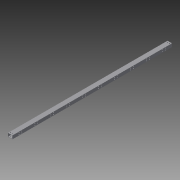
# Autodesk Inventor part: Part1
Saved by Autodesk Inventor 2015 SP1 (Build 190203100, 203)
## iProperties
Created: 2015-03-28
Part Number: Part1
Material: Generic
Document SubType Name: Modeling
Designer: Cyril
Density: 1 g/cm^3
Appearance: Default
Author: Cyril
Autodesk Inventor part; units mm, degrees
ref_plane "YZ Plane" through (0, 0, 0) normal (1, 0, 0) x (0, 1, 0)
ref_plane "XZ Plane" through (0, 0, 0) normal (0, 1, 0) x (-1, 0, 0)
ref_plane "XY Plane" through (0, 0, 0) normal (0, 0, 1) x (1, 0, 0)
sketch "Sketch2" plane through (0, 0, 0) normal (0, 0, 1) x (1, 0, 0)
  line L0 (-18, -13) -> (18, -13)
  line L1 (18, -13) -> (18, 13)
  line L2 (18, 13) -> (-18, 13)
  line L3 (-18, 13) -> (-18, -13)
  line L4 (-17.4388, -13.0791) -> (28.6637, 21.4978) construction
  line L5 (18, -13) -> (-25.5523, 18.4544) construction
  line L6 (-20, -15) -> (20, -15)
  line L7 (20, -15) -> (20, 15)
  line L8 (20, 15) -> (-20, 15)
  line L9 (-20, 15) -> (-20, -15)
  line L10 (-20, -15) -> (20, 15) construction
  line L11 (20, -15) -> (-20, 15) construction
  point P0 (0, 0)
  dimension "d0" = 40
  dimension "d1" = 30
  dimension "d3" = 2
  dimension "d6" = 2
  dimension "d7" = 2
  dimension "d8" = 2
  constraints: 24 end point, 4 parallel, 3 point on line, 2 horizontal, 2 midpoint, 2 perpendicular
  measures "d0" distance of L7.end L8.end
  measures "d1" distance of L8.end L6.start
  measures "d3" distance between parallel lines of L9 L3
  measures "d6" distance between parallel lines of L8 L2
  measures "d7" distance between parallel lines of L7 L1
  measures "d8" distance between parallel lines of L6 L0
extrude "Extrusion1" add sketch "Sketch2" along normal mid plane 1430
sketch "Sketch3" plane through (-20, -15, 715) normal (-1, 0, 0) x (0, 0, 1)
  circle A0 centre (-84, 22.5) radius 3.5
  circle A1 centre (-59, 22.5) radius 3.5
  circle A2 centre (-84, 7.5) radius 3.5
  circle A3 centre (-59, 7.5) radius 3.5
  line L0 (0, 0) -> (-1430, 0) projected
  circle A4 centre (-227, 22.5) radius 3.5
  circle A5 centre (-202, 22.5) radius 3.5
  circle A6 centre (-227, 7.5) radius 3.5
  circle A7 centre (-202, 7.5) radius 3.5
  circle A8 centre (-370, 22.5) radius 3.5
  circle A9 centre (-345, 22.5) radius 3.5
  circle A10 centre (-370, 7.5) radius 3.5
  circle A11 centre (-345, 7.5) radius 3.5
  circle A12 centre (-513, 22.5) radius 3.5
  circle A13 centre (-488, 22.5) radius 3.5
  circle A14 centre (-513, 7.5) radius 3.5
  circle A15 centre (-488, 7.5) radius 3.5
  circle A16 centre (-656, 22.5) radius 3.5
  circle A17 centre (-631, 22.5) radius 3.5
  circle A18 centre (-656, 7.5) radius 3.5
  circle A19 centre (-631, 7.5) radius 3.5
  circle A20 centre (-799, 22.5) radius 3.5
  circle A21 centre (-774, 22.5) radius 3.5
  circle A22 centre (-799, 7.5) radius 3.5
  circle A23 centre (-774, 7.5) radius 3.5
  circle A24 centre (-942, 22.5) radius 3.5
  circle A25 centre (-917, 22.5) radius 3.5
  circle A26 centre (-942, 7.5) radius 3.5
  circle A27 centre (-917, 7.5) radius 3.5
  circle A28 centre (-1085, 22.5) radius 3.5
  circle A29 centre (-1060, 22.5) radius 3.5
  circle A30 centre (-1085, 7.5) radius 3.5
  circle A31 centre (-1060, 7.5) radius 3.5
  circle A32 centre (-1228, 22.5) radius 3.5
  circle A33 centre (-1203, 22.5) radius 3.5
  circle A34 centre (-1228, 7.5) radius 3.5
  circle A35 centre (-1203, 7.5) radius 3.5
  circle A36 centre (-1371, 22.5) radius 3.5
  circle A37 centre (-1346, 22.5) radius 3.5
  circle A38 centre (-1371, 7.5) radius 3.5
  circle A39 centre (-1346, 7.5) radius 3.5
  line L1 (-1716, 15) -> (286, 15) projected
  dimension "d16" = 143
  constraints: 40 centre point, 3 equal radius, 2 horizontal alignment, 2 vertical alignment, 1 horizontal, 73 other
  measures "d16" distance of A0.centre A4.centre
extrude "Extrusion2" cut sketch "Sketch3" against normal through all
sketch "Sketch4" plane through (-20, 15, 715) normal (0, 1, 0) x (1, 0, 0)
  circle A0 centre (11, 12.5) radius 3.5
  circle A1 centre (29, 12.5) radius 3.5
  line L0 (40, 0) -> (0, 0) projected
  line L1 (0, 0) -> (40, 0) projected
  line L2 (20, 0) -> (20, 1430) construction
  line L3 (0, 1430) -> (40, 1430) projected
  circle A2 centre (11, 1417.5) radius 3.5
  circle A3 centre (29, 1417.5) radius 3.5
  point P0 (20, 715)
  dimension "d23" = 7
  dimension "d24" = 12.5
  dimension "d25" = 18
  dimension "d26" = 12.5
  constraints: 4 centre point, 3 equal radius, 2 end point, 2 horizontal alignment, 2 midpoint, 2 vertical alignment, 1 other
  measures "d23" diameter of A0
  measures "d24" distance from line of L0 A0.centre
  measures "d25" distance of A1.centre A0.centre
  measures "d26" distance from line of L3 A2.centre
extrude "Extrusion3" cut sketch "Sketch4" against normal through all
equation "\"d6\" = d3"
equation "\"d7\" = d3"
equation "\"d26\" = d24"
body "Solid1"
